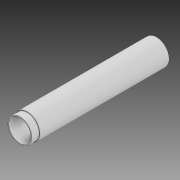
# Autodesk Inventor part: LASER
Saved by Autodesk Inventor 2020 (Build 240168000, 168)
## iProperties
Created: 2020-09-30
Part Number: LASER
Material: Generic
Document SubType Name: Modeling
Designer: DDeGo
Density: 1 g/cm^3
Appearance: Default
Author: DDeGo
Autodesk Inventor part; units mm, degrees
ref_plane "YZ Plane" through (0, 0, 0) normal (1, 0, 0) x (0, 1, 0)
ref_plane "XZ Plane" through (0, 0, 0) normal (0, 1, 0) x (-1, 0, 0)
ref_plane "XY Plane" through (0, 0, 0) normal (0, 0, 1) x (1, 0, 0)
sketch "Sketch1" plane through (0, 0, 0) normal (1, 0, 0) x (0, 1, 0)
  line L0 (0, 0) -> (6.1, 0) construction
  line L1 (6.6, 0) -> (6.6, -4)
  line L2 (6.6, -4) -> (6.95, -4)
  line L3 (6.95, -4) -> (6.95, -74.9)
  line L4 (6.95, -74.9) -> (0, -74.9) construction
  line L5 (0, -74.9) -> (0, -15)
  arc A0 (2.25, -76.9) -> (6.95, -74.9) centre (0, -65.09) ccw
  line L6 (2.25, -76.9) -> (2.25, -75.4)
  line L7 (2.25, -75.4) -> (0, -75.4)
  line L8 (0, -75.4) -> (0, -74.9)
  line L9 (6.1, 0) -> (6.1, -15)
  line L10 (6.1, -15) -> (0, -15)
  line L11 (6.1, 0) -> (6.6, 0)
  line L12 (0, -15) -> (0, 0) construction
  dimension "d0" = 6.95
  dimension "d1" = 6.6
  dimension "d2" = 4
  dimension "d4" = 76.9
  dimension "d5" = 2.25
  dimension "d6" = 1.5
  dimension "d7" = 2
  dimension "d9" = 0.5
  dimension "d10" = 15
  constraints: 26 end point, 13 perpendicular, 2 horizontal, 2 point on circle, 2 vertical, 1 centre point, 1 point on line
  measures "d0" distance between parallel lines of L5 L3
  measures "d1" distance between parallel lines of L5 L1
  measures "d2" distance of L1.start L1.end
  measures "d4" distance from line of L0 L6.start
  measures "d5" distance between parallel lines of L8 L6
  measures "d6" distance of L6.start L6.end
  measures "d7" distance from line of L4 L6.start
  measures "d9" distance between parallel lines of L9 L1
  measures "d10" distance of L0.end L9.end
revolve "Revolution1" add sketch "Sketch1" angle 360 about axis through (0, 0, -74.9) along (0, 0, 1)
body "Solid1"
